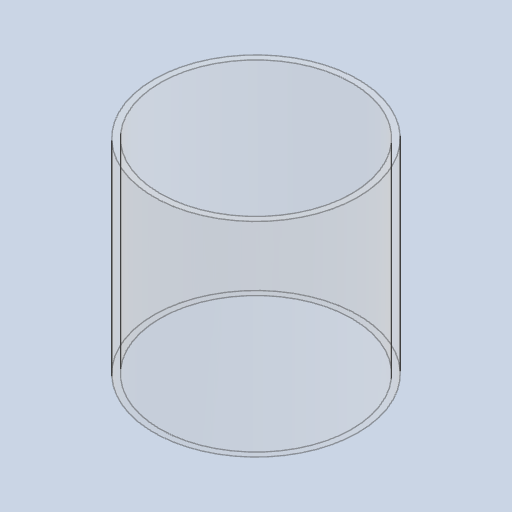
# Autodesk Inventor part: Chasis
Saved by Autodesk Inventor 2024.3 (Build 283343000, 343)
## iProperties
Created: 2024-12-19
Part Number: Chasis
Material: Policarbonato, ahumado
Document SubType Name: Modeling
Designer: Usuario
Density: 1.2 g/cm^3
Appearance: Policarbonato - Claro
Mass: 109.704 g
Surface Area: 627.753 cm^2
Volume: 91.4203 cm^3
Author: Usuario
Autodesk Inventor part; units mm, degrees
ref_plane "YZ Plane" through (0, 0, 0) normal (1, 0, 0) x (0, 1, 0)
ref_plane "XZ Plane" through (0, 0, 0) normal (0, 1, 0) x (-1, 0, 0)
ref_plane "XY Plane" through (0, 0, 0) normal (0, 0, 1) x (1, 0, 0)
sketch "Boceto1" plane through (0, 0, 0) normal (0, 1, 0) x (-1, 0, 0)
  circle A0 centre (0, 0) radius 50
  circle A1 centre (0, 0) radius 47
  dimension "De" = 100
  dimension "Di" = 94
  constraints: 2 centre point, 2 coincident
  measures "De" diameter of A0
  measures "Di" diameter of A1
extrude "Extrusión1" add sketch "Boceto1" along normal blind 100
